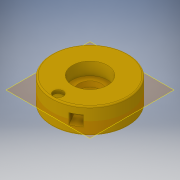
# Autodesk Inventor part: BasePaletasTop
Saved by Autodesk Inventor 2019 (Build 230136000, 136)
## iProperties
Created: 2019-12-12
Part Number: BasePaletasTop
Material: Generic
Document SubType Name: Modeling
Designer: Sergio
Density: 1 g/cm^3
Appearance: Gold
Author: Sergio
Autodesk Inventor part; units mm, degrees
ref_plane "XY Plane" through (0, 0, 0) normal (0, 0, 1) x (1, 0, 0)
sketch "Sketch3" plane through (0, 0, 0) normal (1, 0, 0) x (0, 1, 0)
  line L0 (63.5252, 0) -> (0, 0) construction
  line L1 (0, -8) -> (0, -27)
  line L2 (0, -27) -> (18, -27)
  line L3 (18, -27) -> (18, -12.4)
  line L4 (9, -8) -> (9, -12.4)
  line L5 (9, -12.4) -> (18, -12.4)
  line L6 (9, -8) -> (5, -8)
  line L7 (5, -8) -> (5, 0)
  line L8 (0, -8) -> (0, 0)
  line L9 (5, 0) -> (0, 0)
  dimension "d15" = 18
  dimension "d18" = 9
  dimension "d32" = 27
  dimension "d33" = 12.4
  dimension "d54" = 4
  dimension "d56" = 8
  constraints: 20 end point, 3 perpendicular, 2 horizontal, 2 parallel, 1 coincident, 1 collinear, 1 point on line, 1 vertical
  measures "d15" distance between parallel lines of L3 L1
  measures "d18" distance of L1.start L4.start
  measures "d32" distance between parallel lines of L0 L2
  measures "d33" distance between parallel lines of L0 L5
  measures "d54" distance of L4.start L6.end
  measures "d56" distance of L6.end L7.end
revolve "Revolution1" add sketch "Sketch3" angle 360 about axis through (0, 63.5252, 0) along (0, -1, 0)
fillet "Fillet2" radius 1 2 edges at (0, 18, 27) (0, 0, 27)
ref_plane "Work Plane2" through (-27, 9, 0) normal (1, 0, 0) x (0, 1, 0)
sketch "Sketch4" plane through (-27, 9, 0) normal (1, 0, 0) x (0, 1, 0)
  line L0 (-9, 0) -> (10.8256, 0) construction
  line L1 (-3.75, 3.75) -> (3.75, 3.75)
  line L2 (3.75, 3.75) -> (3.75, -3.75)
  line L3 (3.75, -3.75) -> (-3.75, -3.75)
  line L4 (-3.75, -3.75) -> (-3.75, 3.75)
  line L5 (-3.75, 3.75) -> (3.75, -3.75) construction
  line L6 (3.75, 3.75) -> (-3.75, -3.75) construction
  line L7 (9, 26) -> (9, -26) projected
  point P0 (0, 0)
  dimension "d21" = 7.5
  dimension "d22" = 7.5
  dimension "d55" = 9
  constraints: 14 end point, 2 horizontal, 2 midpoint, 2 parallel, 1 perpendicular, 1 point on line
  measures "d21" distance of L2.end L3.end
  measures "d22" distance of L1.end L2.end
  measures "d55" distance from line of L7 point (0, 0)
extrude "Extrusion3" cut sketch "Sketch4" along normal blind 10
pattern_circular "Circular Pattern2" count 3 over 360 about axis through (0, 13.5, 0) along (0, -1, 0) of "Extrusion3"
sketch "Sketch9" plane through (0, 18, 0) normal (0, 1, 0) x (1, 0, 0)
  circle A0 centre (0, -22.4737) radius 3.5
  point P0 (0, 0)
  dimension "d57" = 7
  constraints: 1 centre point
  measures "d57" diameter of A0
extrude "Extrusion7" cut sketch "Sketch9" against normal blind 2.4
ref_plane "Work Plane4" through (0, 9, 0) normal (0, 1, 0) x (-1, 0, 0)
body "Solid2"
